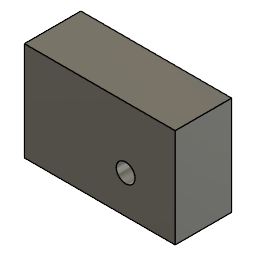
replay (Autodesk Fusion 360 design; units mm, degrees)
Autodesk Fusion 360 part; units mm, degrees
sketch "草图1" plane through (0, 0, 0) normal (0, 0, 1) x (1, 0, 0)
  line L0 (74, -6) -> (74, 36)
  line L1 (74, 36) -> (10, 36)
  line L2 (10, 36) -> (10, -6)
  line L3 (10, -6) -> (74, -6)
extrude "拉伸1" add sketch "草图1" along normal blind 24
sketch "草图2" plane through (0, 0, 24) normal (0, 0, 1) x (1, 0, 0)
  line L0 (10, -6) -> (74, -6)
  line L1 (74, -6) -> (74, 36)
  line L2 (74, 36) -> (10, 36)
  line L3 (10, 36) -> (10, -6)
  circle A0 centre (53, 10) radius 4
extrude "拉伸2" cut sketch "草图2" against normal through all contours A0
